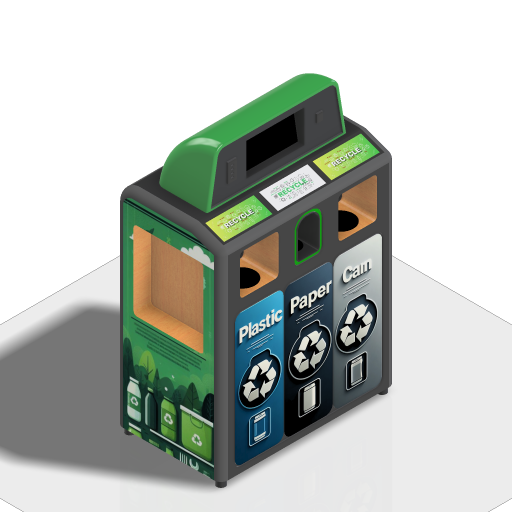
# Autodesk Inventor part: CARCASA_V1
Saved by Autodesk Inventor 2024.1 (Build 281209000, 209)
## iProperties
Created: 2024-04-15
Part Number: CARCASA_V1
Material: Acetal Resin, Black
Document SubType Name: Modeling
Designer: Niler
Density: 1.425 g/cm^3
Appearance: Smooth - Black
Mass: 8112 g
Surface Area: 76616.3 cm^2
Volume: 7652.83 cm^3
Author: Niler
Autodesk Inventor part; units mm, degrees
ref_plane "YZ Plane" through (0, 0, 0) normal (1, 0, 0) x (0, 1, 0)
ref_plane "XZ Plane" through (0, 0, 0) normal (0, 1, 0) x (-1, 0, 0)
ref_plane "XY Plane" through (0, 0, 0) normal (0, 0, 1) x (1, 0, 0)
sketch "Sketch1" plane through (0, 0, 0) normal (0, 1, 0) x (-1, 0, 0)
  line L0 (-300, 500) -> (300, 500)
  line L1 (300, 500) -> (300, -500)
  line L2 (300, -500) -> (-300, -500)
  line L3 (-300, -500) -> (-300, 500)
  line L4 (-300, 500) -> (300, -500) construction
  line L5 (300, 500) -> (-300, -500) construction
  point P0 (0, 0)
  dimension "d0" = 600
  dimension "d1" = 1000
  constraints: 12 end point, 2 midpoint, 2 parallel, 1 horizontal, 1 perpendicular
  measures "d0" distance of L1.end L2.end
  measures "d1" distance of L0.end L1.end
extrude "Extrusion1" add sketch "Sketch1" along normal blind 1200
chamfer "Chamfer1" distance 60 angle 70 1 edges at (300, 1200, 0) measured on face at (300, 1199.5, 0)
fillet "Fillet1" radius 40 10 edges at (300, 570, 500) (-300, 600, 500) (-300, 600, -500) (300, 570, -500) (217.5757, 1170, 500) (217.5757, 1170, -500) (-82.4243, 1200, 500) (-82.4243, 1200, -500) (135.1514, 1200, 0) (300, 1140, 0)
sketch "Sketch3" plane through (-260, 0, 500) normal (0, 0, 1) x (1, 0, 0)
  line L0 (0, 0) -> (0, 1160) projected
  line L1 (0, 0) -> (520, 0) projected
  line L2 (520, 1111.9917) -> (520, 0) projected
  line L3 (388.0983, 1160) -> (520, 1111.9917) projected
  line L4 (0, 1160) -> (388.0983, 1160) projected
  line L5 (80, 1040) -> (440, 1040)
  line L6 (460, 1020) -> (460, 610)
  line L7 (440, 590) -> (80, 590)
  line L8 (60, 610) -> (60, 1020)
  arc A0 (80, 1040) -> (60, 1020) centre (80, 1020) ccw
  arc A1 (460, 1020) -> (440, 1040) centre (440, 1020) ccw
  arc A2 (440, 590) -> (460, 610) centre (440, 610) ccw
  arc A3 (60, 610) -> (80, 590) centre (80, 610) ccw
  point P0 (260, 0)
  dimension "d9" = 20
  dimension "d10" = 60
  dimension "d11" = 60
  dimension "d12" = 120
  dimension "d13" = 450
  constraints: 8 end point, 8 point on circle, 8 tangent, 4 centre point, 3 equal radius, 2 parallel, 1 horizontal, 1 perpendicular
  measures "d9" radius of A0
  measures "d10" distance between parallel lines of L2 L6
  measures "d11" distance between parallel lines of L0 L8
  measures "d12" distance between parallel lines of L4 L5
  measures "d13" distance between parallel lines of L7 L5
extrude "Extrusion2" cut sketch "Sketch3" against normal blind 100 contours L5 A1 L6 A2 L7 A3 L8 A0
sketch "Sketch4" plane through (300, 0, 460) normal (1, 0, 0) x (0, 0, -1)
  line L0 (0, 0) -> (0, 1111.9917) projected
  line L1 (0, 0) -> (920, 0) projected
  line L2 (920, 1111.9917) -> (920, 0) projected
  line L3 (0, 1111.9917) -> (920, 1111.9917) projected
  line L4 (450, 1081.9917) -> (470, 1081.9917)
  line L5 (520, 1031.9917) -> (520, 891.9917)
  line L6 (510, 881.9917) -> (410, 881.9917)
  line L7 (400, 891.9917) -> (400, 1031.9917)
  arc A0 (450, 1081.9917) -> (400, 1031.9917) centre (450, 1031.9917) ccw
  arc A1 (520, 1031.9917) -> (470, 1081.9917) centre (470, 1031.9917) ccw
  arc A2 (400, 891.9917) -> (410, 881.9917) centre (410, 891.9917) ccw
  arc A3 (510, 881.9917) -> (520, 891.9917) centre (510, 891.9917) ccw
  point P0 (460, 0)
  point P1 (460, 881.9917)
  point P2 (460, 1111.9917)
  point P3 (520, 961.9917)
  dimension "d16" = 150
  dimension "d17" = 200
  dimension "d18" = 120
  dimension "d19" = 50
  dimension "d20" = 10
  constraints: 8 end point, 8 point on circle, 8 tangent, 4 centre point, 3 midpoint, 2 equal radius, 2 parallel, 1 horizontal, 1 perpendicular, 1 vertical alignment
  measures "d16" distance from line of L3 point (520, 961.992)
  measures "d17" distance between parallel lines of L6 L4
  measures "d18" distance between parallel lines of L5 L7
  measures "d19" radius of A0
  measures "d20" radius of A2
extrude "Extrusion3" cut sketch "Sketch4" against normal blind 200 contours L4 A1 L5 A3 L6 A2 L7 A0
sketch "Sketch5" plane through (300, 0, 460) normal (1, 0, 0) x (0, 0, -1)
  arc A0 (510, 881.9917) -> (520, 891.9917) centre (510, 891.9917) ccw projected
  line L0 (510, 881.9917) -> (410, 881.9917) projected
  arc A1 (400, 891.9917) -> (410, 881.9917) centre (410, 891.9917) ccw projected
  line L1 (400, 891.9917) -> (400, 1031.9917) projected
  arc A2 (450, 1081.9917) -> (400, 1031.9917) centre (450, 1031.9917) ccw projected
  line L2 (450, 1081.9917) -> (470, 1081.9917) projected
  arc A3 (520, 1031.9917) -> (470, 1081.9917) centre (470, 1031.9917) ccw projected
  line L3 (520, 1031.9917) -> (520, 891.9917) projected
  line L4 (0, 0) -> (0, 1111.9917) projected
  line L5 (0, 0) -> (920, 0) projected
  line L6 (920, 1111.9917) -> (920, 0) projected
  line L7 (0, 1111.9917) -> (920, 1111.9917) projected
  line L8 (0, 0) -> (0, 1111.9917) projected
  line L9 (920, 1111.9917) -> (920, 0) projected
  line L10 (0, 800) -> (920, 800)
  line L11 (920, 800) -> (920, 0)
  line L12 (920, 0) -> (0, 0)
  line L13 (0, 0) -> (0, 800)
  line L14 (320, 800) -> (320, 0)
  line L15 (460, 800) -> (460, 644.3838)
  line L16 (600, 800) -> (600, 0)
  line L17 (40, 795) -> (40, 40)
  line L18 (40, 40) -> (880, 40)
  line L19 (880, 40) -> (880, 795)
  line L20 (317.5, 800) -> (317.5, 0)
  line L21 (322.5, 800) -> (322.5, 0)
  line L22 (597.5, 800) -> (597.5, 0)
  line L23 (602.5, 800) -> (602.5, 0)
  line L24 (0, 0) -> (920, 0) projected
  line L25 (40, 795) -> (880, 795)
  line L26 (35, 35) -> (35, 800)
  line L27 (35, 800) -> (885, 800)
  line L28 (885, 800) -> (885, 35)
  line L29 (885, 35) -> (35, 35)
  point P0 (460, 0)
  point P1 (0, 800)
  point P2 (602.5, 40)
  point P3 (602.5, 795)
  point P4 (317.5, 40)
  point P5 (317.5, 795)
  point P6 (597.5, 795)
  point P7 (597.5, 40)
  point P8 (322.5, 40)
  point P9 (322.5, 795)
  dimension "d23" = 800
  dimension "d26" = 2.5
  dimension "d27" = 2.5
  dimension "d28" = 2.5
  dimension "d29" = 2.5
  dimension "d30" = 5
  dimension "d33" = 40
  dimension "d34" = 280
  dimension "d35" = 5
  constraints: 38 end point, 8 parallel, 7 point on line, 3 perpendicular, 2 symmetric about line, 1 horizontal, 1 midpoint, 1 vertical, 10 other
  measures "d23" distance between parallel lines of L12 L10
  measures "d26" distance between parallel lines of L14 L20
  measures "d27" distance between parallel lines of L14 L21
  measures "d28" distance between parallel lines of L16 L22
  measures "d29" distance between parallel lines of L16 L23
  measures "d30" distance between parallel lines of L10 L25
  measures "d33" distance between parallel lines of L4 L17
  measures "d34" distance between parallel lines of L17 L14
  measures "d35" distance between parallel lines of L17 L26
extrude "Extrusion4" cut sketch "Sketch5" against normal blind 5 contours L10 L20 L25 L17 L18 L29 L26 | L20 L18 L14 L29 | L10 L14 L25 L20 | L14 L18 L21 L29 | L20 L25 L14 L18 | L10 L21 L25 L14 | L21 L18 L22 L29 | L14 L25 L21 L18 | L28 L29 L23 L18 L19 L25 L10 | L10 L15 L25 L21 | L22 L18 L16 L29 | L23 L25 L16 L10 | L10 L22 L25 L15 | L16 L18 L23 L29 | L22 L25 L16 L18 | L16 L25 L22 L10 | L23 L18 L16 L25
fillet "Fillet2" radius 40 16 edges at (297.5, 795, 420) (297.5, 800, 425) (297.5, 795, 142.5) (297.5, 795, 137.5) (297.5, 40, 420) (297.5, 35, 425) (297.5, 40, 142.5) (297.5, 40, 137.5) (297.5, 40, -137.5) (297.5, 40, -142.5) (297.5, 40, -420) (297.5, 35, -425) (297.5, 800, -425) (297.5, 795, -420) (297.5, 795, -137.5) (297.5, 795, -142.5)
sketch "Sketch6" plane through (300, 0, 460) normal (1, 0, 0) x (0, 0, -1)
  line L0 (510, 881.9917) -> (410, 881.9917) projected
  arc A0 (510, 881.9917) -> (520, 891.9917) centre (510, 891.9917) ccw projected
  line L1 (520, 1031.9917) -> (520, 891.9917) projected
  arc A1 (520, 1031.9917) -> (470, 1081.9917) centre (470, 1031.9917) ccw projected
  line L2 (450, 1081.9917) -> (470, 1081.9917) projected
  arc A2 (450, 1081.9917) -> (400, 1031.9917) centre (450, 1031.9917) ccw projected
  line L3 (400, 891.9917) -> (400, 1031.9917) projected
  arc A3 (400, 891.9917) -> (410, 881.9917) centre (410, 891.9917) ccw projected
  arc A4 (450, 1101.9917) -> (380, 1031.9917) centre (450, 1031.9917) ccw
  line L4 (450, 1101.9917) -> (470, 1101.9917)
  arc A5 (540, 1031.9917) -> (470, 1101.9917) centre (470, 1031.9917) ccw
  line L5 (540, 1031.9917) -> (540, 891.9917)
  arc A6 (510, 861.9917) -> (540, 891.9917) centre (510, 891.9917) ccw
  line L6 (510, 861.9917) -> (410, 861.9917)
  arc A7 (380, 891.9917) -> (410, 861.9917) centre (410, 891.9917) ccw
  line L7 (380, 891.9917) -> (380, 1031.9917)
  arc A8 (450, 1086.9917) -> (395, 1031.9917) centre (450, 1031.9917) ccw
  line L8 (450, 1086.9917) -> (470, 1086.9917)
  arc A9 (525, 1031.9917) -> (470, 1086.9917) centre (470, 1031.9917) ccw
  line L9 (525, 1031.9917) -> (525, 891.9917)
  arc A10 (510, 876.9917) -> (525, 891.9917) centre (510, 891.9917) ccw
  line L10 (510, 876.9917) -> (410, 876.9917)
  arc A11 (395, 891.9917) -> (410, 876.9917) centre (410, 891.9917) ccw
  line L11 (395, 891.9917) -> (395, 1031.9917)
  point P0 (460, 0)
  dimension "d37" = 20
  dimension "d38" = 5
  constraints: 16 end point, 16 point on circle, 8 centre point, 14 other
  measures "d37" distance between parallel lines of L3 L7
  measures "d38" distance between parallel lines of L3 L11
extrude "Extrusion5" cut sketch "Sketch6" against normal blind 5 contours L4 A5 L5 A6 L6 A7 L7 A4
sketch "Sketch7" plane through (300, 881.9917, 50) normal (0, 1, 0) x (1, 0, 0)
  line L0 (0, 100) -> (0, 0) projected
  line L1 (0, 100) -> (-200, 100) projected
  line L2 (-200, 100) -> (-200, 0) projected
  line L3 (0, 0) -> (-200, 0) projected
  circle A0 centre (-100, 50) radius 50
  line L4 (0, 100) -> (0, 0) projected
  point P0 (-300, 50)
  point P1 (0, 50)
  point P2 (-100, 100)
  constraints: 2 midpoint, 1 centre point, 1 horizontal alignment, 1 tangent, 1 vertical alignment
extrude "Extrusion6" cut sketch "Sketch7" against normal blind 10 contours A0
sketch "Sketch8" plane through (0, 1200, 0) normal (0, 1, 0) x (1, 0, 0)
  line L0 (128.0983, -460) -> (-300, -460) projected
  line L1 (128.0983, 460) -> (128.0983, -460) projected
  line L2 (-300, 460) -> (128.0983, 460) projected
  line L3 (-300, 460) -> (-300, -460) projected
  line L4 (-300, 460) -> (-300, -460) projected
  line L5 (-220, -400) -> (120, -400)
  line L6 (120, -400) -> (120, 400)
  line L7 (120, 400) -> (-220, 400)
  line L8 (-220, 400) -> (-220, -400)
  point P0 (0, 0)
  point P1 (120, 0)
  point P2 (-300, 400)
  point P3 (-300, -400)
  dimension "d43" = 800
  dimension "d63" = 80
  dimension "d81" = 340
  constraints: 8 end point, 1 horizontal, 1 horizontal alignment, 1 midpoint, 1 parallel, 1 perpendicular, 1 vertical, 1 vertical alignment
  measures "d43" distance between parallel lines of L7 L5
  measures "d63" distance between parallel lines of L3 L8
  measures "d81" distance between parallel lines of L6 L8
extrude "Extrusion7" add sketch "Sketch8" along normal blind 300 contours L8 L7 L6 L5
sketch "Sketch9" plane through (-300, 1200, 400) normal (0, 0, 1) x (1, 0, 0)
  line L0 (420, 0) -> (80, 0) projected
  line L1 (420, 0) -> (420, 300) projected
  line L2 (80, 300) -> (420, 300) projected
  circle A0 centre (420, -7.7066) radius 307.7066
  line L3 (80, 300) -> (420, 300) projected
  line L4 (420, 300) -> (329.5855, 0)
  line L5 (80, 0) -> (80, 300) projected
  point P0 (300, -1200)
  point P1 (0, 350)
  point P2 (310.7868, 0)
  point P3 (420, 280.5117)
  point P4 (112.3899, 0)
  point P5 (380, 349.796)
  point P6 (251.4342, 350)
  point P7 (80, 190)
  constraints: 3 point on line, 2 end point, 4 other
extrude "Extrusion8" cut sketch "Sketch9" against normal through all contours A0 L0 L5 L2
sketch "Sketch14" plane through (120, 1200, 400) normal (1, 0, 0) x (0, 0, -1)
  line L0 (800, 0) -> (0, 0) projected
  line L1 (800, 0) -> (800, 300) projected
  line L2 (0, 300) -> (800, 300) projected
  line L3 (0, 0) -> (0, 300) projected
  line L4 (400, 300) -> (400, 206.4643)
  line L5 (0, 0) -> (50, 300)
  line L6 (800, 0) -> (750, 300)
  point P0 (400, -1200)
  dimension "d84" = 50
  constraints: 6 end point, 1 midpoint, 1 point on line, 1 symmetric about line, 1 vertical
  measures "d84" distance from line of L3 L5.end
extrude "Extrusion12" cut sketch "Sketch14" against normal through all contours L6 L2 L1 | L3 L2 L5
fillet "Fillet3" radius 60 2 edges at (-94.8395, 1412.5827, 364.5696) (-94.8395, 1412.5827, -364.5696)
fillet "Fillet4" radius 10 1 edges at (120, 1500, 0)
sketch "Sketch11" plane through (0, 0, 0) normal (0, 0, 1) x (1, 0, 0)
  line L0 (120, 1437.1135) -> (120, 1250)
  line L1 (40, 1437.1135) -> (120, 1437.1135)
  line L2 (120, 1250) -> (72.9932, 1250)
  line L3 (72.9932, 1250) -> (40, 1437.1135)
  line L4 (120, 1200) -> (120, 1448.018) projected
  line L5 (120, 1448.018) -> (120, 1200) projected
  line L6 (120, 1489.832) -> (120, 1448.018) projected
  line L7 (120, 1448.018) -> (120, 1489.832) projected
  point P0 (0, 0)
  dimension "d59" = 50
  dimension "d60" = 190
  dimension "d61" = 80
  dimension "d62" = 100
  constraints: 8 end point, 1 horizontal, 1 perpendicular
  measures "d59" distance of L4.start L0.end
  measures "d60" distance of L2.end L1.start
  measures "d61" distance of L1.start L0.start
  measures "d62" angle of L2 L3
extrude "Extrusion10" cut sketch "Sketch11" along normal mid plane 332
sketch "Sketch12" plane through (120, 1200, 389.8621) normal (1, 0, 0) x (0, 0, -1)
  line L0 (555.8621, 237.1135) -> (555.8621, 50) projected
  line L1 (555.8621, 50) -> (223.8621, 50) projected
  line L2 (223.8621, 50) -> (223.8621, 237.1135) projected
  line L3 (223.8621, 237.1135) -> (555.8621, 237.1135) projected
  line L4 (779.7241, 0) -> (0, 0) projected
  line L5 (90.6664, 289.832) -> (689.0577, 289.832) projected
  line L6 (110.4432, 190.1091) -> (160.4432, 190.1091)
  line L7 (160.4432, 190.1091) -> (160.4432, 84.1091)
  line L8 (160.4432, 84.1091) -> (110.4432, 84.1091)
  line L9 (110.4432, 84.1091) -> (110.4432, 190.1091)
  line L10 (622.9885, 121.9778) -> (649.5251, 121.9778)
  line L11 (649.5251, 121.9778) -> (649.5251, 114.2728)
  line L12 (649.5251, 114.2728) -> (622.9885, 114.2728)
  line L13 (622.9885, 114.2728) -> (622.9885, 121.9778)
  line L14 (619.2396, 175.5308) -> (653.274, 175.5308)
  line L15 (653.274, 175.5308) -> (653.274, 130.0344)
  line L16 (653.274, 130.0344) -> (619.2396, 130.0344)
  line L17 (619.2396, 130.0344) -> (619.2396, 175.5308)
  line L18 (127.9432, 170.1091) -> (142.9432, 170.1091)
  line L19 (142.9432, 170.1091) -> (142.9432, 164.1091)
  line L20 (142.9432, 164.1091) -> (127.9432, 164.1091)
  line L21 (127.9432, 164.1091) -> (127.9432, 170.1091)
  line L22 (142.9432, 150.1091) -> (142.9432, 144.1091)
  line L23 (127.9432, 150.1091) -> (142.9432, 150.1091)
  line L24 (127.9432, 144.1091) -> (127.9432, 150.1091)
  line L25 (142.9432, 144.1091) -> (127.9432, 144.1091)
  line L26 (142.9432, 130.1091) -> (142.9432, 124.1091)
  line L27 (127.9432, 130.1091) -> (142.9432, 130.1091)
  line L28 (127.9432, 124.1091) -> (127.9432, 130.1091)
  line L29 (142.9432, 124.1091) -> (127.9432, 124.1091)
  line L30 (142.9432, 110.1091) -> (142.9432, 104.1091)
  line L31 (127.9432, 110.1091) -> (142.9432, 110.1091)
  line L32 (127.9432, 104.1091) -> (127.9432, 110.1091)
  line L33 (142.9432, 104.1091) -> (127.9432, 104.1091)
  line L34 (105.4432, 195.1091) -> (165.4432, 195.1091)
  line L35 (165.4432, 195.1091) -> (165.4432, 79.1091)
  line L36 (165.4432, 79.1091) -> (105.4432, 79.1091)
  line L37 (105.4432, 79.1091) -> (105.4432, 195.1091)
  line L38 (616.2396, 178.5308) -> (656.274, 178.5308)
  line L39 (656.274, 178.5308) -> (656.274, 127.0344)
  line L40 (656.274, 127.0344) -> (616.2396, 127.0344)
  line L41 (616.2396, 127.0344) -> (616.2396, 178.5308)
  line L42 (0, 0) -> (41.3363, 248.018) projected
  line L43 (738.3878, 248.018) -> (779.7241, 0) projected
  point P0 (389.8621, -1200)
  point P1 (135.4432, 190.1091)
  point P2 (135.4432, 170.1091)
  point P3 (636.2568, 121.9778)
  point P4 (636.2568, 130.0344)
  point P5 (636.2568, 175.5308)
  dimension "d64" = 6
  dimension "d65" = 15
  dimension "d68" = 20
  dimension "d73" = 20
  dimension "d74" = 20
  dimension "d75" = 5
  dimension "d76" = 60
  dimension "d77" = 3
  constraints: 72 end point, 12 parallel, 6 perpendicular, 5 midpoint, 4 horizontal, 3 vertical alignment, 1 vertical, 32 other
  measures "d64" distance of L20.end L18.start
  measures "d65" distance of L18.start L18.end
  measures "d68" distance of L20.start L22.end
  measures "d73" distance from line of L6 point (135.443, 170.109)
  measures "d74" distance between parallel lines of L8 L33
  measures "d75" distance between parallel lines of L9 L37
  measures "d76" distance between parallel lines of L35 L37
  measures "d77" distance between parallel lines of L17 L41
extrude "Extrusion11" cut sketch "Sketch12" against normal blind 10 contours L10 L11 L12 L13 | L18 L19 L20 L21 | L22 L25 L24 L23 | L26 L29 L28 L27 | L30 L33 L32 L31 | L34 L35 L36 L37 | L38 L39 L40 L41
fillet "Fillet5" radius 100 3 edges at (-288.2843, 1188.2843, 488.2843) (-288.2843, 1188.2843, -488.2843) (-300, 1200, 0)
sketch "Sketch13" plane through (-300, 0, -460) normal (-1, 0, 0) x (0, 0, 1)
  arc A0 (602.5, 80) -> (642.5, 40) centre (642.5, 80) ccw projected
  line L0 (602.5, 80) -> (602.5, 755) projected
  arc A1 (642.5, 795) -> (602.5, 755) centre (642.5, 755) ccw projected
  line L1 (642.5, 795) -> (840, 795) projected
  arc A2 (880, 755) -> (840, 795) centre (840, 755) ccw projected
  line L2 (880, 755) -> (880, 80) projected
  arc A3 (840, 40) -> (880, 80) centre (840, 80) ccw projected
  line L3 (840, 40) -> (642.5, 40) projected
  arc A4 (362.5, 795) -> (322.5, 755) centre (362.5, 755) ccw projected
  line L4 (362.5, 795) -> (557.5, 795) projected
  arc A5 (597.5, 755) -> (557.5, 795) centre (557.5, 755) ccw projected
  line L5 (597.5, 755) -> (597.5, 80) projected
  arc A6 (557.5, 40) -> (597.5, 80) centre (557.5, 80) ccw projected
  line L6 (557.5, 40) -> (362.5, 40) projected
  arc A7 (322.5, 80) -> (362.5, 40) centre (362.5, 80) ccw projected
  line L7 (322.5, 80) -> (322.5, 755) projected
  arc A8 (317.5, 755) -> (277.5, 795) centre (277.5, 755) ccw projected
  line L8 (317.5, 755) -> (317.5, 80) projected
  arc A9 (277.5, 40) -> (317.5, 80) centre (277.5, 80) ccw projected
  line L9 (277.5, 40) -> (80, 40) projected
  arc A10 (40, 80) -> (80, 40) centre (80, 80) ccw projected
  line L10 (40, 80) -> (40, 755) projected
  arc A11 (80, 795) -> (40, 755) centre (80, 755) ccw projected
  line L11 (80, 795) -> (277.5, 795) projected
  circle A12 centre (17.6911, 42.1) radius 25
  arc A13 (312.5, 755) -> (277.5, 790) centre (277.5, 755) ccw
  line L12 (312.5, 755) -> (312.5, 80)
  arc A14 (277.5, 45) -> (312.5, 80) centre (277.5, 80) ccw
  line L13 (277.5, 45) -> (80, 45)
  arc A15 (45, 80) -> (80, 45) centre (80, 80) ccw
  line L14 (45, 80) -> (45, 755)
  arc A16 (80, 790) -> (45, 755) centre (80, 755) ccw
  line L15 (80, 790) -> (277.5, 790)
  line L16 (557.5, 790) -> (362.5, 790)
  arc A17 (362.5, 790) -> (327.5, 755) centre (362.5, 755) ccw
  line L17 (327.5, 755) -> (327.5, 80)
  arc A18 (327.5, 80) -> (362.5, 45) centre (362.5, 80) ccw
  line L18 (362.5, 45) -> (557.5, 45)
  arc A19 (557.5, 45) -> (592.5, 80) centre (557.5, 80) ccw
  line L19 (592.5, 80) -> (592.5, 755)
  arc A20 (592.5, 755) -> (557.5, 790) centre (557.5, 755) ccw
  line L20 (840, 790) -> (642.5, 790)
  arc A21 (642.5, 790) -> (607.5, 755) centre (642.5, 755) ccw
  line L21 (607.5, 755) -> (607.5, 80)
  arc A22 (607.5, 80) -> (642.5, 45) centre (642.5, 80) ccw
  line L22 (642.5, 45) -> (840, 45)
  arc A23 (840, 45) -> (875, 80) centre (840, 80) ccw
  line L23 (875, 80) -> (875, 755)
  arc A24 (875, 755) -> (840, 790) centre (840, 755) ccw
  line L24 (70, 1080) -> (850, 1080)
  line L25 (880, 1050) -> (880, 850)
  line L26 (850, 820) -> (70, 820)
  line L27 (40, 850) -> (40, 1050)
  line L28 (0, 1100) -> (920, 1100) projected
  arc A25 (70, 1080) -> (40, 1050) centre (70, 1050) ccw
  arc A26 (40, 850) -> (70, 820) centre (70, 850) ccw
  arc A27 (850, 820) -> (880, 850) centre (850, 850) ccw
  arc A28 (880, 1050) -> (850, 1080) centre (850, 1050) ccw
  line L29 (850, 1075) -> (70, 1075)
  arc A29 (70, 1075) -> (45, 1050) centre (70, 1050) ccw
  line L30 (45, 1050) -> (45, 850)
  arc A30 (45, 850) -> (70, 825) centre (70, 850) ccw
  line L31 (70, 825) -> (850, 825)
  arc A31 (850, 825) -> (875, 850) centre (850, 850) ccw
  line L32 (875, 850) -> (875, 1050)
  arc A32 (875, 1050) -> (850, 1075) centre (850, 1050) ccw
  circle A33 centre (245, 1045) radius 15
  circle A34 centre (675, 1045) radius 15
  circle A35 centre (282.5, 417.5) radius 15
  circle A36 centre (562.5, 417.5) radius 15
  circle A37 centre (845, 417.5) radius 15
  point P0 (460, 0)
  point P1 (460, 1080)
  point P2 (460, 1100)
  point P3 (312.5, 417.5)
  dimension "d82" = 50
  dimension "d87" = 5
  dimension "d88" = 5
  dimension "d89" = 5
  dimension "d90" = 30
  dimension "d91" = 20
  dimension "d92" = 260
  dimension "d93" = 840
  dimension "d94" = 5
  dimension "d95" = 30
  dimension "d96" = 200
  dimension "d97" = 200
  dimension "d98" = 35
  dimension "d99" = 30
  dimension "d100" = 30
  dimension "d101" = 30
  constraints: 40 end point, 40 point on circle, 26 centre point, 8 tangent, 7 equal radius, 4 horizontal alignment, 4 parallel, 3 midpoint, 2 perpendicular, 1 horizontal, 1 vertical alignment, 28 other
  measures "d82" diameter of A12
  measures "d87" distance between parallel lines of L11 L15
  measures "d88" distance between parallel lines of L4 L16
  measures "d89" distance between parallel lines of L1 L20
  measures "d90" radius of A25
  measures "d91" distance between parallel lines of L28 L24
  measures "d92" distance between parallel lines of L24 L26
  measures "d93" distance between parallel lines of L25 L27
  measures "d94" distance between parallel lines of L24 L29
  measures "d95" diameter of A33
  measures "d96" distance from line of L30 A33.centre
  measures "d97" distance from line of L32 A34.centre
  measures "d98" distance from line of L24 A33.centre
  measures "d99" distance from line of L12 A35.centre
  measures "d100" distance from line of L19 A36.centre
  measures "d101" distance from line of L23 A37.centre
extrude "Extrusion13" cut sketch "Sketch13" against normal blind 5 contours L0 A1 L1 A2 L2 A3 L3 A0 | L4 A5 L5 A6 L6 A7 L7 A4 | L8 A9 L9 A10 L10 A11 L11 A8 | L24 A28 L25 A27 L26 A26 L27 A25 | A33 | A34 | A35 | A36 | A37
sketch "Sketch15" plane through (300, 0, 460) normal (1, 0, 0) x (0, 0, -1)
  line L0 (845, 35) -> (75, 35) projected
  arc A0 (35, 75) -> (75, 35) centre (75, 75) ccw projected
  line L1 (35, 75) -> (35, 760) projected
  arc A1 (75, 800) -> (35, 760) centre (75, 760) ccw projected
  line L2 (75, 800) -> (845, 800) projected
  arc A2 (885, 760) -> (845, 800) centre (845, 760) ccw projected
  line L3 (885, 760) -> (885, 75) projected
  arc A3 (845, 35) -> (885, 75) centre (845, 75) ccw projected
  line L4 (0, 0) -> (0, 1111.9917) projected
  line L5 (0, 0) -> (920, 0) projected
  line L6 (920, 1111.9917) -> (920, 0) projected
  line L7 (0, 1111.9917) -> (920, 1111.9917) projected
  arc A4 (450, 1101.9917) -> (380, 1031.9917) centre (450, 1031.9917) ccw projected
  line L8 (450, 1101.9917) -> (470, 1101.9917) projected
  arc A5 (540, 1031.9917) -> (470, 1101.9917) centre (470, 1031.9917) ccw projected
  line L9 (540, 1031.9917) -> (540, 891.9917) projected
  arc A6 (510, 861.9917) -> (540, 891.9917) centre (510, 891.9917) ccw projected
  line L10 (510, 861.9917) -> (410, 861.9917) projected
  arc A7 (380, 891.9917) -> (410, 861.9917) centre (410, 891.9917) ccw projected
  line L11 (380, 891.9917) -> (380, 1031.9917) projected
  line L12 (88.75, 1091.9917) -> (268.75, 1091.9917)
  line L13 (288.75, 1071.9917) -> (288.75, 881.9917)
  line L14 (268.75, 861.9917) -> (88.75, 861.9917)
  line L15 (68.75, 881.9917) -> (68.75, 1071.9917)
  arc A8 (88.75, 1091.9917) -> (68.75, 1071.9917) centre (88.75, 1071.9917) ccw
  arc A9 (288.75, 1071.9917) -> (268.75, 1091.9917) centre (268.75, 1071.9917) ccw
  arc A10 (268.75, 861.9917) -> (288.75, 881.9917) centre (268.75, 881.9917) ccw
  arc A11 (68.75, 881.9917) -> (88.75, 861.9917) centre (88.75, 881.9917) ccw
  arc A12 (277.5, 40) -> (317.5, 80) centre (277.5, 80) ccw projected
  line L16 (317.5, 80) -> (317.5, 755) projected
  arc A13 (317.5, 755) -> (277.5, 795) centre (277.5, 755) ccw projected
  line L17 (277.5, 795) -> (80, 795) projected
  arc A14 (80, 795) -> (40, 755) centre (80, 755) ccw projected
  line L18 (40, 755) -> (40, 80) projected
  arc A15 (40, 80) -> (80, 40) centre (80, 80) ccw projected
  line L19 (80, 40) -> (277.5, 40) projected
  line L20 (460, 1111.9917) -> (460, 815.5453)
  line L21 (831.25, 1091.9917) -> (651.25, 1091.9917)
  line L22 (631.25, 1071.9917) -> (631.25, 881.9917)
  line L23 (651.25, 861.9917) -> (831.25, 861.9917)
  line L24 (851.25, 881.9917) -> (851.25, 1071.9917)
  arc A16 (851.25, 1071.9917) -> (831.25, 1091.9917) centre (831.25, 1071.9917) ccw
  arc A17 (651.25, 1091.9917) -> (631.25, 1071.9917) centre (651.25, 1071.9917) ccw
  arc A18 (631.25, 881.9917) -> (651.25, 861.9917) centre (651.25, 881.9917) ccw
  arc A19 (831.25, 861.9917) -> (851.25, 881.9917) centre (831.25, 881.9917) ccw
  point P0 (460, 0)
  point P1 (288.75, 976.9917)
  point P2 (380, 961.9917)
  point P3 (178.75, 861.9917)
  point P4 (178.75, 795)
  point P5 (631.25, 976.9917)
  point P6 (741.25, 861.9917)
  point P7 (460, 861.9917)
  dimension "d104" = 20
  dimension "d105" = 230
  dimension "d106" = 220
  constraints: 18 end point, 16 point on circle, 14 symmetric about line, 8 centre point, 8 tangent, 6 midpoint, 3 equal radius, 2 parallel, 2 perpendicular, 1 horizontal, 1 horizontal alignment, 1 vertical alignment, 4 other
  measures "d104" radius of A8
  measures "d105" distance between parallel lines of L14 L12
  measures "d106" distance between parallel lines of L13 L15
extrude "Extrusion14" cut sketch "Sketch15" against normal blind 200 contours L12 A9 L13 A10 L14 A11 L15 A8 | A16 L24 A19 L23 A18 L22 A17 L21
sketch "Sketch16" plane through (300, 861.9917, 371.25) normal (0, 1, 0) x (1, 0, 0)
  line L0 (0, 180) -> (0, 0) projected
  line L1 (0, 180) -> (-200, 180) projected
  line L2 (-200, 180) -> (-200, 0) projected
  line L3 (0, 0) -> (-200, 0) projected
  line L4 (0, 742.5) -> (0, 562.5) projected
  line L5 (0, 742.5) -> (-200, 742.5) projected
  line L6 (-200, 742.5) -> (-200, 562.5) projected
  line L7 (0, 562.5) -> (-200, 562.5) projected
  circle A0 centre (-100, 90) radius 75
  circle A1 centre (-100, 652.5) radius 75
  point P0 (-300, 371.25)
  point P1 (-200, 90)
  point P2 (-100, 180)
  point P3 (-100, 742.5)
  point P4 (-200, 652.5)
  dimension "d109" = 150
  constraints: 4 midpoint, 2 centre point, 2 horizontal alignment, 2 vertical alignment, 1 equal radius
  measures "d109" diameter of A0
extrude "Extrusion15" cut sketch "Sketch16" against normal blind 10 contours A0 | A1
ref_plane "Work Plane1" through (400, 80, 137.5) normal (1, 0, 0) x (0, 0, -1)
sketch "Sketch18" plane through (400, 80, 137.5) normal (1, 0, 0) x (0, 0, -1)
  arc A0 (-45, -40) -> (-5, 0) centre (-45, 0) ccw projected
  line L0 (-5, 0) -> (-5, 675) projected
  arc A1 (-5, 675) -> (-45, 715) centre (-45, 675) ccw projected
  line L1 (-45, 715) -> (-242.5, 715) projected
  arc A2 (-242.5, 715) -> (-282.5, 675) centre (-242.5, 675) ccw projected
  line L2 (-282.5, 675) -> (-282.5, 0) projected
  arc A3 (-282.5, 0) -> (-242.5, -40) centre (-242.5, 0) ccw projected
  line L3 (-242.5, -40) -> (-45, -40) projected
  arc A4 (275, 675) -> (235, 715) centre (235, 675) ccw projected
  line L4 (235, 715) -> (40, 715) projected
  arc A5 (40, 715) -> (0, 675) centre (40, 675) ccw projected
  line L5 (0, 675) -> (0, 0) projected
  arc A6 (0, 0) -> (40, -40) centre (40, 0) ccw projected
  line L6 (40, -40) -> (235, -40) projected
  arc A7 (235, -40) -> (275, 0) centre (235, 0) ccw projected
  line L7 (275, 0) -> (275, 675) projected
  arc A8 (320, 715) -> (280, 675) centre (320, 675) ccw projected
  line L8 (280, 675) -> (280, 0) projected
  arc A9 (280, 0) -> (320, -40) centre (320, 0) ccw projected
  line L9 (320, -40) -> (517.5, -40) projected
  arc A10 (517.5, -40) -> (557.5, 0) centre (517.5, 0) ccw projected
  line L10 (557.5, 0) -> (557.5, 675) projected
  arc A11 (557.5, 675) -> (517.5, 715) centre (517.5, 675) ccw projected
  line L11 (517.5, 715) -> (320, 715) projected
  line L12 (-288.3745, 715.0946) -> (10.7375, 715.0946) construction
  line L13 (10.7375, 715.0946) -> (10.7375, -39.9054) construction
  line L14 (10.7375, -39.9054) -> (-288.3745, -39.9054) construction
  line L15 (-288.3745, -39.9054) -> (-288.3745, 715.0946) construction
  line L16 (-2.7299, 714.971) -> (288.1308, 714.971) construction
  line L17 (288.1308, 714.971) -> (288.1308, -40.029) construction
  line L18 (288.1308, -40.029) -> (-2.7299, -40.029) construction
  line L19 (-2.7299, -40.029) -> (-2.7299, 714.971) construction
  line L20 (267.2111, 714.9795) -> (558.0718, 714.9795) construction
  line L21 (558.0718, 714.9795) -> (558.0718, -40.0205) construction
  line L22 (558.0718, -40.0205) -> (267.2111, -40.0205) construction
  line L23 (267.2111, -40.0205) -> (267.2111, 714.9795) construction
  point P0 (137.5, -80)
  dimension "d142" = 755
  dimension "d159" = 755
  constraints: 6 other
  measures "d142" distance between parallel lines of L14 L12
  measures "d159" distance of L18.end L16.start
decal "Decal2"
decal "Decal3"
decal "Decal4"
ref_plane "Work Plane2" through (400, 0, 460) normal (1, 0, 0) x (0, 0, -1)
ref_plane "Work Plane3" through (260, 0, -809) normal (0, 0, -1) x (-1, 0, 0)
ref_plane "Work Plane4" through (-260, 0, 925) normal (0, 0, 1) x (1, 0, 0)
sketch "Sketch21" plane through (-260, 0, 925) normal (0, 0, 1) x (1, 0, 0)
  arc A0 (60, 1160) -> (0, 1100) centre (60, 1100) ccw projected
  line L0 (0, 0) -> (0, 1100) projected
  line L1 (0, 0) -> (520, 0) projected
  line L2 (520, 1111.9917) -> (520, 0) projected
  line L3 (388.0983, 1160) -> (520, 1111.9917) projected
  line L4 (60, 1160) -> (388.0983, 1160) projected
  arc A1 (440, 590) -> (460, 610) centre (440, 610) ccw projected
  line L5 (440, 590) -> (80, 590) projected
  arc A2 (60, 610) -> (80, 590) centre (80, 610) ccw projected
  line L6 (60, 610) -> (60, 1020) projected
  arc A3 (80, 1040) -> (60, 1020) centre (80, 1020) ccw projected
  line L7 (80, 1040) -> (440, 1040) projected
  arc A4 (460, 1020) -> (440, 1040) centre (440, 1020) ccw projected
  line L8 (460, 1020) -> (460, 610) projected
  line L9 (0, 1160) -> (520, 1160) construction
  line L10 (520, 1160) -> (520, -520.8082) construction
  line L11 (520, -520.8082) -> (0, -520.8082) construction
  line L12 (0, -520.8082) -> (0, 1160) construction
  line L13 (520, 1113.4579) -> (396.7513, 1160)
  point P0 (260, 0)
  dimension "d217" = 520
  constraints: 2 end point, 2 point on line, 2 other
  measures "d217" distance of L10.end L11.end
decal "Decal7"
sketch "Sketch22" plane through (260, 0, -809) normal (0, 0, -1) x (-1, 0, 0)
  line L0 (-0.0569, 1158.9773) -> (519.9431, 1158.9773) construction
  line L1 (519.9431, 1158.9773) -> (519.9431, -521.8309) construction
  line L2 (519.9431, -521.8309) -> (-0.0569, -521.8309) construction
  line L3 (-0.0569, -521.8309) -> (-0.0569, 1158.9773) construction
  arc A0 (520, 1100) -> (460, 1160) centre (460, 1100) ccw projected
  line L4 (131.9017, 1160) -> (460, 1160) projected
  line L5 (0, 1111.9917) -> (131.9017, 1160) projected
  line L6 (0, 0) -> (0, 1111.9917) projected
  line L7 (0, 0) -> (520, 0) projected
  line L8 (520, 1100) -> (520, 0) projected
  point P0 (260, 0)
  dimension "d226" = 520
  constraints: 2 other
  measures "d226" distance of L0.start L0.end
decal "Decal8"
ref_plane "Work Plane5" through (867.75, 1200, 389.8621) normal (1, 0, 0) x (0, 0, -1)
sketch "Sketch25" plane through (120, 1200, 389.8621) normal (1, 0, 0) x (0, 0, -1)
  line L0 (649.5251, 121.9778) -> (649.5251, 114.2728) projected
  line L1 (649.5251, 114.2728) -> (622.9885, 114.2728) projected
  line L2 (622.9885, 114.2728) -> (622.9885, 121.9778) projected
  line L3 (622.9885, 121.9778) -> (649.5251, 121.9778) projected
  line L4 (656.274, 178.5308) -> (656.274, 127.0344) projected
  line L5 (656.274, 127.0344) -> (616.2396, 127.0344) projected
  line L6 (616.2396, 127.0344) -> (616.2396, 178.5308) projected
  line L7 (616.2396, 178.5308) -> (656.274, 178.5308) projected
  line L8 (165.4432, 195.1091) -> (165.4432, 79.1091) projected
  line L9 (165.4432, 79.1091) -> (105.4432, 79.1091) projected
  line L10 (105.4432, 79.1091) -> (105.4432, 195.1091) projected
  line L11 (105.4432, 195.1091) -> (165.4432, 195.1091) projected
  line L12 (555.8621, 237.1135) -> (555.8621, 50) projected
  line L13 (555.8621, 50) -> (223.8621, 50) projected
  line L14 (223.8621, 50) -> (223.8621, 237.1135) projected
  line L15 (223.8621, 237.1135) -> (555.8621, 237.1135) projected
  line L16 (0, 0) -> (41.3363, 248.018) projected
  line L17 (779.7241, 0) -> (0, 0) projected
  line L18 (738.3878, 248.018) -> (779.7241, 0) projected
  spline S0 degree 7 poles (689.0577, 289.832) (693.6675, 289.832) (698.4551, 289.3359) (703.3368, 288.2749) (708.1987, 286.5987) (712.8958, 284.2976) (717.2905, 281.4227) (723.2745, 276.3784) (725.1692, 274.5733) (726.9483, 272.6572) (728.6008, 270.6439) (730.1181, 268.5484) (731.4947, 266.3869) (733.9591, 261.9682) (735.0474, 259.7112) (735.9906, 257.4204) (736.7886, 255.1114) (737.4446, 252.8004) (737.9642, 250.501) (738.3584, 248.193) (738.3635, 248.163) (738.3685, 248.1334) (738.3733, 248.1046) (738.3782, 248.0757) (738.383, 248.0469) (738.3878, 248.0181) knots 0 0 0 0 0 0 0 0 0.498507 0.498507 0.498507 0.498507 0.498507 0.498507 0.74818 0.74818 0.74818 0.74818 0.74818 0.74818 0.997373 0.997373 0.997373 0.997373 0.997373 0.997373 1 1 1 1 1 1 1 1 weights 1 1 1 1 1 1 1 1 1 1 1 1 1 1 1 1 1 1 1 1 1 1 1 1 1 1
  line L19 (90.6664, 289.832) -> (689.0577, 289.832) projected
  spline S1 degree 7 poles (41.3363, 248.0181) (41.3411, 248.0469) (41.346, 248.0757) (41.3508, 248.1046) (41.3557, 248.1334) (41.3607, 248.163) (41.3658, 248.193) (41.76, 250.501) (42.2796, 252.8004) (42.9355, 255.1114) (43.7335, 257.4204) (44.6767, 259.7112) (45.765, 261.9682) (48.2294, 266.3869) (49.606, 268.5484) (51.1233, 270.6439) (52.7758, 272.6572) (54.5549, 274.5733) (56.4496, 276.3785) (62.4337, 281.4227) (66.8284, 284.2976) (71.5254, 286.5987) (76.3873, 288.2749) (81.269, 289.3359) (86.0566, 289.832) (90.6664, 289.832) knots 0 0 0 0 0 0 0 0 0.002627 0.002627 0.002627 0.002627 0.002627 0.002627 0.25182 0.25182 0.25182 0.25182 0.25182 0.25182 0.501493 0.501493 0.501493 0.501493 0.501493 0.501493 1 1 1 1 1 1 1 1 weights 1 1 1 1 1 1 1 1 1 1 1 1 1 1 1 1 1 1 1 1 1 1 1 1 1 1
  line L20 (728.5238, 246.374) -> (767.9195, 10)
  line L21 (767.9195, 10) -> (11.8046, 10)
  line L22 (11.8046, 10) -> (51.2003, 246.374)
  line L23 (90.6664, 279.832) -> (689.0577, 279.832)
  spline S2 degree 5 poles (689.0577, 279.832) (694.6772, 279.8319) (700.2967, 278.8447) (705.6847, 276.8691) (715.5477, 271.1055) (722.856, 262.3243) (725.6963, 257.3227) (727.5981, 251.9297) (728.5238, 246.3741) knots 0 0 0 0 0 0 0.499432 0.499432 0.499432 1 1 1 1 1 1
  spline S3 degree 5 poles (51.2003, 246.3741) (52.1261, 251.9297) (54.0278, 257.3227) (56.8681, 262.3243) (64.1764, 271.1055) (74.0395, 276.8691) (79.4274, 278.8447) (85.0469, 279.8319) (90.6664, 279.832) knots 0 0 0 0 0 0 0.500568 0.500568 0.500568 1 1 1 1 1 1
  point P0 (389.8621, -1200)
  dimension "d257" = 10
  constraints: 8 end point, 3 parallel, 10 other
  measures "d257" distance between parallel lines of L19 L23
extrude "Extrusion16" cut sketch "Sketch25" against normal blind 10 contours L20 L21 L22 S3 L23 S2
ref_plane "Work Plane6" through (315.0652, 1263.2822, 460) normal (0.3420201, 0.9396926, 0) x (0.9396926, -0.3420201, 0)
sketch "Sketch26" plane through (315.0652, 1263.2822, 460) normal (0.3420201, 0.9396926, 0) x (0.9396926, -0.3420201, 0)
  line L0 (-125.3584, 627.0487) -> (-125.3584, 903.7404) construction
  line L1 (-125.3584, 903.7404) -> (-10.3584, 903.7404) construction
  line L2 (-10.3584, 903.7404) -> (-10.3584, 627.0487) construction
  line L3 (-10.3584, 627.0487) -> (-125.3584, 627.0487) construction
  line L4 (-126.4328, 15.1099) -> (-126.4328, 291.8017) construction
  line L5 (-126.4328, 291.8017) -> (-11.4328, 291.8017) construction
  line L6 (-11.4328, 291.8017) -> (-11.4328, 15.1099) construction
  line L7 (-11.4328, 15.1099) -> (-126.4328, 15.1099) construction
  line L8 (-125.8083, 321.8936) -> (-125.8083, 598.0662) construction
  line L9 (-125.8083, 598.0662) -> (-10.8083, 598.0662) construction
  line L10 (-10.8083, 598.0662) -> (-10.8083, 321.8936) construction
  line L11 (-10.8083, 321.8936) -> (-125.8083, 321.8936) construction
  point P0 (136.0035, 460)
  dimension "d325" = 115
  dimension "d338" = 115
  dimension "d343" = 115
  constraints: 6 other
  measures "d325" distance of L5.start L5.end
  measures "d338" distance of L2.end L0.start
  measures "d343" distance of L8.end L9.end
decal "Decal10"
decal "Decal11"
decal "Decal12"
sketch "Sketch27" plane through (0, 0, 0) normal (0, -1, 0) x (1, 0, 0)
  arc A0 (-260, 500) -> (-300, 460) centre (-260, 460) ccw projected
  line L0 (-300, -460) -> (-300, 460) projected
  arc A1 (-300, -460) -> (-260, -500) centre (-260, -460) ccw projected
  line L1 (260, -500) -> (-260, -500) projected
  arc A2 (260, -500) -> (300, -460) centre (260, -460) ccw projected
  line L2 (300, 460) -> (300, -460) projected
  arc A3 (300, 460) -> (260, 500) centre (260, 460) ccw projected
  line L3 (-260, 500) -> (260, 500) projected
  circle A4 centre (-260, 460) radius 25
  circle A5 centre (260, 460) radius 25
  circle A6 centre (260, -460) radius 25
  circle A7 centre (-260, -460) radius 25
  point P0 (0, 0)
  dimension "d355" = 50
  constraints: 4 centre point, 4 coincident, 3 equal radius
  measures "d355" diameter of A4
extrude "Extrusion17" add sketch "Sketch27" along normal blind 40 contours A4 | A5 | A6 | A7
body "Solid1"
